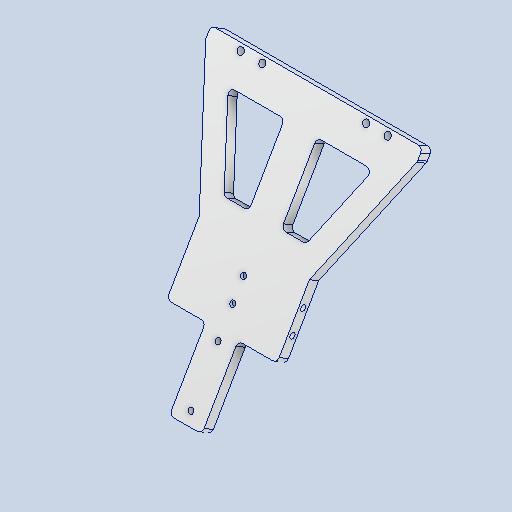
# Autodesk Inventor part: belt_liner_v5_Plate_5
Saved by Autodesk Inventor 2025.2 (Build 292293000, 293)
## iProperties
Created: 2025-02-23
Part Number: belt_liner_v5_Plate_5
Material: アルミニウム 6061
Document SubType Name: Modeling
Designer: haruy
Density: 2.7 g/cm^3
Appearance: アルミニウム - フラット
Author: haruy
Autodesk Inventor part; units mm, degrees
ref_plane "YZ Plane" through (0, 0, 0) normal (1, 0, 0) x (0, 1, 0)
ref_plane "XZ Plane" through (0, 0, 0) normal (0, 1, 0) x (-1, 0, 0)
ref_plane "XY Plane" through (0, 0, 0) normal (0, 0, 1) x (1, 0, 0)
derived "belt_liner_v5_Sketch_Base.ipt"
sketch "スケッチ1" plane through (300, 0, 0) normal (1, 0, 0) x (0, 1, 0)
  circle A0 centre (0, 0) radius 22.36
  circle A1 centre (742.4003, -428.625) radius 23.875 construction
  line L0 (0, 0) -> (0, -985.832)
  line L1 (0, 0) -> (742.4003, -428.625)
  line L2 (-48.7433, -24.4258) -> (-56.2433, -37.4162)
  line L3 (-56.2433, -37.4162) -> (725.7777, -488.9162)
  line L4 (725.7777, -488.9162) -> (733.2777, -475.9258)
  line L5 (733.2777, -475.9258) -> (-48.7433, -24.4258)
  line L6 (-44.1225, 123.2584) -> (-44.1225, 123.2584)
  line L7 (0, -985.832) -> (0, 0)
  circle A2 centre (0, 0) radius 12.5
  circle A3 centre (0, 0) radius 15
  line L8 (0, 0) -> (0, 0)
  circle A4 centre (0, 0) radius 24.06 construction
  line L9 (0, 0) -> (0, 0)
  line L10 (0, 0) -> (0, 0)
  line L11 (-48.7433, -24.4258) -> (-46.2433, -20.0957)
  circle A5 centre (742.4003, -428.625) radius 5
  line L12 (733.2777, -475.9258) -> (707.2969, -460.9258)
  line L13 (707.2969, -460.9258) -> (709.7969, -456.5957)
  line L14 (709.7969, -456.5957) -> (735.7777, -471.5957)
  line L15 (735.7777, -471.5957) -> (733.2777, -475.9258)
  circle A6 centre (738.0702, -426.125) radius 5.1
  line L16 (742.4003, -428.625) -> (509.0943, -293.9257)
  circle A7 centre (759.7208, -438.625) radius 5.1
  line L17 (740.6202, -421.7083) -> (762.2708, -434.2083)
  line L18 (735.5202, -430.5417) -> (757.1708, -443.0417)
  circle A8 centre (742.4003, -428.625) radius 22.175 construction
  circle A9 centre (738.0702, -426.125) radius 10.1 construction
  circle A10 centre (759.7208, -438.625) radius 10.1 construction
  line L19 (743.1202, -417.3781) -> (764.7708, -429.8781) construction
  line L20 (733.0202, -434.8719) -> (754.6708, -447.3719) construction
  line L21 (743.1202, -417.3781) -> (730.6598, -410.1842) construction
  line L22 (729.3233, -421.075) -> (734.3733, -412.3281) construction
  line L23 (764.7708, -429.8781) -> (770.9335, -433.4362) construction
  line L24 (770.9335, -433.4362) -> (771.2695, -433.6302)
  line L25 (754.6708, -447.3719) -> (764.7708, -429.8781)
  line L26 (764.7708, -429.8781) -> (773.431, -434.8781)
  line L27 (773.431, -434.8781) -> (763.331, -452.3719)
  line L28 (763.331, -452.3719) -> (754.6708, -447.3719) construction
  circle A11 centre (725.8674, -468.7607) radius 1.5
  circle A12 centre (0, 0) radius 30
  circle A13 centre (742.4003, -428.625) radius 6 construction
  circle A14 centre (0, 0) radius 24.06 construction
  circle A15 centre (0, 0) radius 24.06
  circle A16 centre (742.4003, -428.625) radius 24.06
  line L29 (754.4303, -407.7884) -> (12.03, 20.8366)
  circle A17 centre (725.8592, -419.075) radius 4
  circle A18 centre (725.8592, -419.075) radius 1.5
  circle A19 centre (742.4003, -428.625) radius 18.525 construction
  circle A20 centre (748.9869, -417.4167) radius 4
  line L30 (737.4369, -437.4219) -> (742.4869, -428.675)
  circle A21 centre (748.9869, -417.4167) radius 1.5
  line L31 (734.3733, -412.3281) -> (737.8233, -406.3526) construction
  line L32 (737.8233, -406.3526) -> (776.881, -428.9026)
  line L33 (773.431, -434.8781) -> (776.881, -428.9026)
  line L34 (737.8233, -406.3526) -> (723.6503, -415.7402)
  line L35 (720.8233, -435.7974) -> (759.881, -458.3474)
  line L36 (720.8233, -435.7974) -> (721.8667, -418.8295)
  line L37 (763.331, -452.3719) -> (759.881, -458.3474)
  circle A22 centre (735.9869, -439.9333) radius 4
  circle A23 centre (735.9869, -439.9333) radius 1.5
  circle A24 centre (717.2072, -463.7607) radius 1.5
  circle A25 centre (742.4003, -428.625) radius 34.06
  circle A26 centre (742.4869, -428.675) radius 8.5
  line L38 (-57.9836, -13.421) -> (-72.9836, -13.421)
  line L39 (-72.9836, -13.421) -> (-72.9836, -278.421)
  line L40 (-72.9836, -278.421) -> (-57.9836, -278.421)
  line L41 (-57.9836, -278.421) -> (-57.9836, -13.421)
  line L42 (327.0164, -263.421) -> (-72.9836, -263.421)
  line L43 (-72.9836, -263.421) -> (-72.9836, -278.421)
  line L44 (-72.9836, -278.421) -> (327.0164, -278.421)
  line L45 (327.0164, -278.421) -> (327.0164, -263.421)
  line L46 (297.0164, -263.421) -> (297.0164, -278.421)
  line L47 (327.0164, -278.421) -> (361.1893, -278.421)
  line L48 (361.1893, -278.421) -> (368.6893, -265.4306)
  line L49 (-207.9836, 176.579) -> (-227.9836, 176.579)
  line L50 (-227.9836, 176.579) -> (-227.9836, -413.421)
  line L51 (-227.9836, -413.421) -> (-207.9836, -413.421)
  line L52 (-207.9836, -413.421) -> (-207.9836, 176.579)
  line L53 (-51.4069, -263.5692) -> (-53.919, -273.2486)
  line L54 (-53.919, -273.2486) -> (703.31, -469.7727)
  line L55 (703.31, -469.7727) -> (705.822, -460.0934)
  line L56 (705.822, -460.0934) -> (-51.4069, -263.5692)
  circle A27 centre (0, 0) radius 24.06
  line L57 (1412.7204, 281.579) -> (-606.6364, 281.579)
  line L58 (1185.5776, -518.421) -> (-909.402, -518.421)
  line L59 (9.7721, 46.9258) -> (885.3238, -458.5742)
  line L60 (885.3238, -458.5742) -> (892.8238, -445.5838)
  line L61 (892.8238, -445.5838) -> (17.2721, 59.9162)
  line L62 (17.2721, 59.9162) -> (9.7721, 46.9258)
  line L63 (32.4276, 51.1662) -> (872.4722, -433.8338)
  line L64 (872.4722, -433.8338) -> (876.2222, -427.3386)
  line L65 (876.2222, -427.3386) -> (36.1776, 57.6614)
  line L66 (36.1776, 57.6614) -> (32.4276, 51.1662)
  line L67 (36.1776, 57.6614) -> (94.8941, 23.7614)
  line L68 (94.8941, 23.7614) -> (97.6441, 28.5245)
  line L69 (97.6441, 28.5245) -> (38.9276, 62.4245)
  line L70 (38.9276, 62.4245) -> (36.1776, 57.6614)
  circle A28 centre (218.0519, 108.5407) radius 120
  line L71 (77.0164, 123.579) -> (57.0164, 123.579)
  line L72 (57.0164, 123.579) -> (57.0164, 103.579)
  line L73 (57.0164, 103.579) -> (77.0164, 103.579)
  line L74 (77.0164, 103.579) -> (77.0164, 123.579)
  line L75 (218.0519, 108.5407) -> (186.9936, 224.4518)
  line L76 (218.0519, 108.5407) -> (102.1408, 77.4824)
  line L77 (218.0519, 108.5407) -> (158.0519, 4.6177)
  line L78 (189.9936, 229.648) -> (99.1408, 72.2863)
  line L79 (99.1408, 72.2863) -> (93.9447, 75.2863)
  line L80 (93.9447, 75.2863) -> (184.7975, 232.648)
  line L81 (184.7975, 232.648) -> (189.9936, 229.648)
  line L82 (184.7975, 232.648) -> (181.7975, 227.4518)
  line L83 (181.7975, 227.4518) -> (177.4674, 229.9518)
  line L84 (177.4674, 229.9518) -> (180.4674, 235.148)
  line L85 (180.4674, 235.148) -> (184.7975, 232.648)
  line L86 (93.9447, 75.2863) -> (96.9447, 80.4824)
  line L87 (96.9447, 80.4824) -> (92.6146, 82.9824)
  line L88 (92.6146, 82.9824) -> (89.6146, 77.7863)
  line L89 (89.6146, 77.7863) -> (93.9447, 75.2863)
  line L90 (77.0164, 123.579) -> (117.0164, 123.579)
  line L91 (117.0164, 123.579) -> (117.0164, 103.579)
  line L92 (117.0164, 103.579) -> (77.0164, 103.579)
  line L93 (77.0164, 103.579) -> (77.0164, 123.579)
  circle A29 centre (218.0519, 108.5407) radius 132.0681
  line L94 (103.6776, 174.5748) -> (38.9276, 62.4245)
  line L95 (32.4276, 51.1662) -> (11.6951, 15.2564)
  line L96 (11.6951, 15.2564) -> (20.3553, 10.2564)
  line L97 (20.3553, 10.2564) -> (41.0878, 46.1662)
  line L98 (41.0878, 46.1662) -> (32.4276, 51.1662)
  line L99 (152.0179, -5.8336) -> (158.0519, 4.6177)
  line L100 (152.0179, -5.8336) -> (20.3553, 10.2564)
  line L101 (74.8121, 3.6014) -> (78.3121, 9.6636)
  line L102 (78.3121, 9.6636) -> (92.5711, 1.4312)
  line L103 (181.7975, 227.4518) -> (154.2911, 210.1998)
  line L104 (96.9447, 80.4824) -> (98.1322, 112.9297)
  line L105 (99.1408, 72.2863) -> (116.3929, 44.7799)
  line L106 (-324.9836, 281.579) -> (-324.9836, -518.421)
  line L107 (1175.0164, 281.579) -> (1175.0164, -518.421)
  line L108 (17.2721, 59.9162) -> (9.7721, 46.9258)
  line L109 (9.7721, 46.9258) -> (-3.2183, 54.4258)
  line L110 (-3.2183, 54.4258) -> (4.2817, 67.4162)
  line L111 (4.2817, 67.4162) -> (17.2721, 59.9162)
  line L112 (-3.2183, 54.4258) -> (-5.7183, 50.0957)
  line L113 (-5.7183, 50.0957) -> (22.4276, 33.8457)
  line L114 (22.4276, 33.8457) -> (24.9276, 38.1758)
  line L115 (24.9276, 38.1758) -> (-3.2183, 54.4258)
  line L116 (-48.7433, -24.4258) -> (-46.2433, -20.0957)
  line L117 (-46.2433, -20.0957) -> (5.7183, -50.0957)
  line L118 (5.7183, -50.0957) -> (3.2183, -54.4258)
  line L119 (3.2183, -54.4258) -> (-48.7433, -24.4258)
  line L120 (789.6086, -403.313) -> (798.2689, -408.313)
  line L121 (798.2689, -408.313) -> (785.0364, -431.2324)
  line L122 (785.0364, -431.2324) -> (776.3761, -426.2324)
  line L123 (776.3761, -426.2324) -> (789.6086, -403.313)
  line L124 (885.3238, -458.5742) -> (882.8238, -462.9043)
  line L125 (882.8238, -462.9043) -> (856.843, -447.9043)
  line L126 (856.843, -447.9043) -> (859.343, -443.5742)
  line L127 (859.343, -443.5742) -> (885.3238, -458.5742)
  line L128 (7.6071, 48.1758) -> (11.9372, 45.6758)
  line L129 (11.9372, 45.6758) -> (19.4372, 58.6662)
  line L130 (19.4372, 58.6662) -> (15.1071, 61.1662)
  line L131 (15.1071, 61.1662) -> (7.6071, 48.1758)
  line L132 (19.4372, 58.6662) -> (14.4372, 50.0059)
  line L133 (14.4372, 50.0059) -> (24.8295, 44.0059)
  line L134 (24.8295, 44.0059) -> (29.8295, 52.6662)
  line L135 (29.8295, 52.6662) -> (19.4372, 58.6662)
  line L136 (931.2231, -485.0742) -> (935.5533, -487.5742)
  line L137 (935.5533, -487.5742) -> (951.5533, -459.8614)
  line L138 (951.5533, -459.8614) -> (947.2231, -457.3614)
  line L139 (947.2231, -457.3614) -> (931.2231, -485.0742)
  line L140 (944.4731, -462.1245) -> (934.9731, -478.579)
  line L141 (934.9731, -478.579) -> (919.3847, -469.579)
  line L142 (919.3847, -469.579) -> (928.8847, -453.1245)
  line L143 (928.8847, -453.1245) -> (944.4731, -462.1245)
  line L144 (924.1347, -461.3518) -> (939.7231, -470.3518)
  line L145 (926.6347, -457.0216) -> (921.6347, -465.6819)
  line L146 (921.6347, -465.6819) -> (882.6635, -443.1819)
  line L147 (882.6635, -443.1819) -> (887.6635, -434.5216)
  line L148 (887.6635, -434.5216) -> (926.6347, -457.0216)
  line L149 (888.9135, -432.3566) -> (881.4135, -445.347)
  line L150 (881.4135, -445.347) -> (874.4853, -441.347)
  line L151 (874.4853, -441.347) -> (881.9853, -428.3566)
  line L152 (881.9853, -428.3566) -> (888.9135, -432.3566)
  line L153 (31.0795, 54.8313) -> (23.5795, 41.8409)
  line L154 (23.5795, 41.8409) -> (30.5077, 37.8409)
  line L155 (30.5077, 37.8409) -> (38.0077, 50.8313)
  line L156 (38.0077, 50.8313) -> (31.0795, 54.8313)
  line L157 (16.9372, 54.3361) -> (27.3295, 48.3361)
  circle A30 centre (4.192, 47.2607) radius 1.25
  circle A31 centre (12.8522, 42.2607) radius 1.25
  line L158 (17.2721, 59.9162) -> (9.7721, 46.9258)
  line L159 (885.3238, -458.5742) -> (882.8238, -462.9043)
  line L160 (882.8238, -462.9043) -> (933.0533, -491.9043)
  line L161 (933.0533, -491.9043) -> (935.5533, -487.5742)
  line L162 (935.5533, -487.5742) -> (885.3238, -458.5742)
  line L163 (375.0164, 281.579) -> (375.0164, -518.421)
  line L164 (38.9276, 62.4245) -> (41.4276, 66.7546)
  line L165 (41.4276, 66.7546) -> (100.1441, 32.8546)
  line L166 (100.1441, 32.8546) -> (97.6441, 28.5245)
  line L167 (97.6441, 28.5245) -> (38.9276, 62.4245)
  line L168 (97.7242, 18.6633) -> (115.0447, 8.6633)
  line L169 (115.0447, 8.6633) -> (117.5447, 12.9934)
  line L170 (117.5447, 12.9934) -> (100.2242, 22.9934)
  line L171 (100.2242, 22.9934) -> (97.7242, 18.6633)
  line L172 (116.2947, 10.8284) -> (98.9742, 20.8284)
  line L173 (327.0164, -263.421) -> (335.2086, -263.421)
  line L174 (335.2086, -263.421) -> (342.7086, -250.4306)
  line L175 (-48.7433, -24.4258) -> (-56.2433, -37.4162)
  line L176 (-56.2433, -37.4162) -> (-77.8939, -24.9162)
  line L177 (-77.8939, -24.9162) -> (-70.3939, -11.9258)
  line L178 (-70.3939, -11.9258) -> (-48.7433, -24.4258)
  line L179 (-207.9836, -73.421) -> (-72.9836, -73.421)
  line L180 (-72.9836, -73.421) -> (-72.9836, -93.421)
  line L181 (-72.9836, -93.421) -> (-207.9836, -93.421)
  line L182 (-207.9836, -93.421) -> (-207.9836, -73.421)
  line L183 (-72.9836, -198.421) -> (-207.9836, -198.421)
  line L184 (-207.9836, -198.421) -> (-207.9836, -218.421)
  line L185 (-207.9836, -218.421) -> (-72.9836, -218.421)
  line L186 (-72.9836, -218.421) -> (-72.9836, -198.421)
  line L187 (-227.9836, -118.421) -> (-207.9836, -118.421)
  circle A32 centre (-30.1728, -32.2607) radius 1.25
  circle A33 centre (-12.8522, -42.2607) radius 1.25
  line L188 (-5.7183, 50.0957) -> (-46.2433, -20.0957)
  circle A34 centre (44.6769, 5.3827) radius 15
  circle A35 centre (17.6769, -41.3827) radius 15
  circle A36 centre (44.6769, 5.3827) radius 22
  circle A37 centre (17.6769, -41.3827) radius 22
  circle A38 centre (31.1769, -18) radius 3
  line L189 (44.6769, 5.3827) -> (17.6769, -41.3827)
  circle A39 centre (26.7448, 25.5678) radius 3
  circle A40 centre (-8.77, -35.9456) radius 3
  circle A41 centre (866.7533, -450.7393) radius 1.25
  circle A42 centre (875.4135, -455.7393) radius 1.25
  circle A43 centre (994.8767, -339.9593) radius 120
  line L190 (278.0519, 212.4638) -> (1054.8767, -236.0362)
  line L191 (-207.9836, -118.421) -> (1175.0164, -118.421)
  line L192 (-227.9836, -283.421) -> (-207.9836, -283.421)
  line L193 (-72.9836, -68.421) -> (-92.9836, -68.421)
  line L194 (-92.9836, -68.421) -> (-92.9836, -88.421)
  line L195 (-92.9836, -88.421) -> (-72.9836, -88.421)
  line L196 (-72.9836, -88.421) -> (-72.9836, -68.421)
  line L197 (-72.9836, -218.421) -> (-92.9836, -218.421)
  line L198 (-92.9836, -218.421) -> (-92.9836, -238.421)
  line L199 (-92.9836, -238.421) -> (-72.9836, -238.421)
  line L200 (-72.9836, -238.421) -> (-72.9836, -218.421)
  circle A44 centre (-28.7272, -34.6374) radius 15
  line L201 (-92.9836, 143.579) -> (-112.9836, 143.579)
  line L202 (-112.9836, 143.579) -> (-112.9836, -340.421)
  line L203 (-112.9836, -340.421) -> (-92.9836, -340.421)
  line L204 (-92.9836, -340.421) -> (-92.9836, 143.579)
  line L205 (-98.6706, -321.2466) -> (-92.9836, -340.421)
  line L206 (-92.9836, -340.421) -> (762.3277, -86.7414)
  line L207 (762.3277, -86.7414) -> (756.6407, -67.567)
  line L208 (756.6407, -67.567) -> (-98.6706, -321.2466)
  line L209 (297.0164, -278.421) -> (282.0164, -278.421)
  line L210 (282.0164, -278.421) -> (282.0164, -293.421)
  line L211 (282.0164, -293.421) -> (297.0164, -293.421)
  line L212 (297.0164, -293.421) -> (297.0164, -278.421)
  line L213 (282.0164, -293.421) -> (267.0164, -293.421)
  line L214 (267.0164, -293.421) -> (267.0164, -210.9924)
  line L215 (267.0164, -210.9924) -> (282.0164, -210.9924)
  line L216 (282.0164, -210.9924) -> (282.0164, -293.421)
  line L217 (947.2231, -457.3614) -> (854.3308, -403.73)
  circle A45 centre (257.8891, 85.5407) radius 120
  line L218 (-189.9836, 176.579) -> (-189.9836, -384.0126)
  point P0 (730.6598, -410.1842)
  point P1 (-65.4836, -23.421)
  point P2 (-65.4836, -270.921)
  point P3 (317.0164, -270.921)
  point P4 (307.0164, -270.921)
  point P5 (347.6105, -261.921)
  point P6 (356.2707, -266.921)
  point P7 (-42.9836, -270.921)
  point P8 (694.8867, -462.421)
  point P9 (57.0164, 113.579)
  point P10 (782.9924, -414.7727)
  point P11 (931.9289, -465.8518)
  point P12 (274.5164, -220.9924)
extrude "押し出し1" add sketch "スケッチ1" against normal blind 51 contours L59 L124 L125 L126
sketch "スケッチ2" plane through (249, 885.3238, -458.5742) normal (0, 0.5, 0.8660254) x (1, 0, 0)
  line L0 (51, -30) -> (0, -30) projected
  line L1 (18, -30) -> (33, -30)
  line L2 (33, -30) -> (33, -63.5)
  line L3 (33, -63.5) -> (18, -63.5)
  line L4 (18, -63.5) -> (18, -30)
  line L5 (0, -30) -> (0, 0) projected
  circle A0 centre (25.5, -58.5) radius 1.25
  circle A1 centre (25.5, -33.5) radius 1.25
  circle A2 centre (25.5, -20) radius 1.25
  circle A3 centre (25.5, -10) radius 1.25
  line L6 (34.5, 58) -> (74.5, 58)
  line L7 (74.5, 58) -> (74.5, 53)
  line L8 (74.5, 53) -> (34.5, 53)
  line L9 (34.5, 53) -> (34.5, 58)
  line L10 (51, 0) -> (0, 0) projected
  line L11 (54.5, 58) -> (54.5, 53)
  circle A4 centre (49.5, 55.5) radius 1.5
  circle A5 centre (59.5, 55.5) radius 1.5
  line L12 (51, 0) -> (74.5, 53)
  line L13 (25.5, -63.5) -> (25.5, -30)
  line L14 (16.5, 58) -> (-23.5, 58)
  line L15 (-23.5, 58) -> (-23.5, 53)
  line L16 (-23.5, 53) -> (16.5, 53)
  line L17 (16.5, 53) -> (16.5, 58)
  circle A6 centre (1.5, 55.5) radius 1.5
  circle A7 centre (-8.5, 55.5) radius 1.5
  line L18 (0, 0) -> (-23.5, 53)
  line L19 (16.5, 58) -> (34.5, 58)
  line L20 (-23.5, 43) -> (26.5, 43)
  line L21 (26.5, 43) -> (26.5, 58)
  line L22 (9.1417, 4.0534) -> (-14.3583, 57.0534)
  line L23 (51, -40) -> (-10, -40)
  line L24 (-10, -40) -> (-10, 10)
  line L25 (-10, 10) -> (44.495, 10)
  line L26 (44.495, 10) -> (65.3583, 57.0534)
  line L27 (74.5, 43) -> (24.5, 43)
  line L28 (24.5, 43) -> (24.5, 58)
  line L29 (18, 43) -> (33, 43)
  line L30 (33, 43) -> (33, 10)
  line L31 (33, 10) -> (18, 10)
  line L32 (18, 10) -> (18, 43)
  point P0 (-249, -996)
  point P1 (-8.1271, 43)
  point P2 (26.5, 43)
  point P3 (59.1271, 43)
  point P4 (6.505, 10)
  point P5 (18, 10)
  point P6 (33, 43)
  dimension "d3" = 15
  dimension "d4" = 18
  dimension "d5" = 33.5
  dimension "d6" = 2.5
  dimension "d7" = 2.5
  dimension "d8" = 7.5
  dimension "d9" = 7.5
  dimension "d10" = 5
  dimension "d11" = 25
  dimension "d12" = 2.5
  dimension "d13" = 13.5
  dimension "d14" = 7.5
  dimension "d15" = 2.5
  dimension "d16" = 10
  dimension "d17" = 7.5
  dimension "d23" = 5
  dimension "d24" = 53
  dimension "d25" = 40
  dimension "d26" = 21.5
  dimension "d27" = 3
  dimension "d28" = 3
  dimension "d29" = 15
  dimension "d30" = 10
  dimension "d31" = 2.5
  dimension "d32" = 2.5
  dimension "d33" = 10
  dimension "d34" = 10
  dimension "d35" = 10
  dimension "d36" = 10
  dimension "d39" = 7.5
  dimension "d40" = 7.5
  constraints: 60 end point, 8 centre point, 7 parallel, 6 symmetric about line, 4 horizontal, 4 midpoint, 3 perpendicular, 3 point on line, 7 other
  measures "d3" distance of L2.end L3.end
  measures "d4" distance between parallel lines of L5 L4
  measures "d5" distance between parallel lines of L3 L0
  measures "d6" diameter of A0
  measures "d7" diameter of A1
  measures "d8" distance from line of A0.centre L4
  measures "d9" distance from line of A1.centre L4
  measures "d10" distance from line of A0.centre L3
  measures "d11" distance of A0.centre A1.centre
  measures "d12" diameter of A2
  measures "d13" distance of A1.centre A2.centre
  measures "d14" distance from line of L4 A2.centre
  measures "d15" diameter of A3
  measures "d16" distance of A2.centre A3.centre
  measures "d17" distance from line of A3.centre L4
  measures "d23" distance of L6.end L7.end
  measures "d24" distance between parallel lines of L10 L8
  measures "d25" distance between parallel lines of L7 L9
  measures "d26" distance between parallel lines of L2 L11
  measures "d27" diameter of A4
  measures "d28" diameter of A5
  measures "d29" distance from line of A4.centre L9
  measures "d30" distance of A5.centre A4.centre
  measures "d31" distance from line of A4.centre L6
  measures "d32" distance from line of A5.centre L6
  measures "d33" distance between parallel lines of L16 L20
  measures "d34" distance between parallel lines of L18 L22
  measures "d35" distance between parallel lines of L10 L25
  measures "d36" distance between parallel lines of L8 L27
  measures "d39" distance between parallel lines of L13 L32
  measures "d40" distance between parallel lines of L13 L30
extrude "押し出し2" add sketch "スケッチ2" against normal blind 5 contours L2 L23 L13 A1 L0 | L13 A1 L23 L4 L0 | L2 L3 L13 A0 L23 | L13 A0 L3 L4 L23
extrude "押し出し3" cut sketch "スケッチ2" against normal blind 5 contours A2 | A3
fillet "フィレット1" radius 2 6 edges at (282, 829.0812, -428.9893) (282, 858.093, -445.7393) (300, 858.093, -445.7393) (267, 858.093, -445.7393) (249, 858.093, -445.7393) (267, 829.0812, -428.9893)
extrude "押し出し4" add sketch "スケッチ2" against normal blind 5 contours L18 L25 L26 L27 L12 L10 | L18 L20 L22 L25 | L27 L26 L8 L12 | L18 L16 L22 L20 | L8 L11 L6 L7 | L27 L21 L19 L9 L8 L26 | L15 L14 L17 L16 | L22 L16 L17 L19 L28 L20 | L32 L20 L27 L30 L25 | L11 L8 L9 L6 | L20 L28 L19 L21
fillet "フィレット2" radius 2 12 edges at (282, 892.7341, -465.7393) (293.495, 892.7341, -465.7393) (308.1271, 921.3129, -482.2393) (282, 921.3129, -482.2393) (323.5, 929.9731, -487.2393) (323.5, 934.3033, -489.7393) (267, 892.7341, -465.7393) (267, 921.3129, -482.2393) (255.505, 892.7341, -465.7393) (240.8729, 921.3129, -482.2393) (225.5, 934.3033, -489.7393) (225.5, 929.9731, -487.2393)
equation "\"d9\" = d8"
equation "\"d14\" = d8"
equation "\"d17\" = d9"
equation "\"d32\" = d31"
